Autodesk Fusion 360 part; units mm, degrees
(part 9 of 40)
  line L3796 (254.4894, 100.1276) -> (254.5417, 99.976) construction
  line L3797 (254.5417, 99.976) -> (254.593, 99.8239) construction
  line L3798 (254.593, 99.8239) -> (254.6434, 99.6712) construction
  line L3799 (254.6434, 99.6712) -> (254.6928, 99.518) construction
  line L3800 (254.6928, 99.518) -> (254.7414, 99.3642) construction
  line L3801 (254.7414, 99.3642) -> (254.789, 99.21) construction
  line L3802 (254.789, 99.21) -> (254.8357, 99.0553) construction
  line L3803 (254.8357, 99.0553) -> (254.8815, 98.9001) construction
  line L3804 (254.8815, 98.9001) -> (254.9265, 98.7444) construction
  line L3805 (254.9265, 98.7444) -> (254.9706, 98.5882) construction
  line L3806 (254.9706, 98.5882) -> (255.0138, 98.4316) construction
  line L3807 (255.0138, 98.4316) -> (255.0561, 98.2745) construction
  line L3808 (255.0561, 98.2745) -> (255.0976, 98.117) construction
  line L3809 (255.0976, 98.117) -> (255.1383, 97.9591) construction
  line L3810 (255.1383, 97.9591) -> (255.1781, 97.8007) construction
  line L3811 (255.1781, 97.8007) -> (255.217, 97.6419) construction
  line L3812 (255.217, 97.6419) -> (255.2551, 97.4827) construction
  line L3813 (255.2551, 97.4827) -> (255.2924, 97.3231) construction
  line L3814 (255.2924, 97.3231) -> (255.3289, 97.1631) construction
  line L3815 (255.3289, 97.1631) -> (255.3646, 97.0027) construction
  line L3816 (255.3646, 97.0027) -> (255.3994, 96.8419) construction
  line L3817 (255.3994, 96.8419) -> (255.4335, 96.6807) construction
  line L3818 (255.4335, 96.6807) -> (255.4667, 96.5191) construction
  line L3819 (255.4667, 96.5191) -> (255.4992, 96.3572) construction
  line L3820 (255.4992, 96.3572) -> (255.5308, 96.1949) construction
  line L3821 (255.5308, 96.1949) -> (255.5617, 96.0323) construction
  line L3822 (255.5617, 96.0323) -> (255.5917, 95.8693) construction
  line L3823 (255.5917, 95.8693) -> (255.621, 95.706) construction
  line L3824 (255.621, 95.706) -> (255.6495, 95.5423) construction
  line L3825 (255.6495, 95.5423) -> (255.6773, 95.3783) construction
  line L3826 (255.6773, 95.3783) -> (255.7043, 95.2139) construction
  line L3827 (255.7043, 95.2139) -> (255.7304, 95.0492) construction
  line L3828 (255.7304, 95.0492) -> (255.7559, 94.8842) construction
  line L3829 (255.7559, 94.8842) -> (255.7806, 94.7189) construction
  line L3830 (255.7806, 94.7189) -> (255.8045, 94.5533) construction
  line L3831 (255.8045, 94.5533) -> (255.8276, 94.3874) construction
  line L3832 (255.8276, 94.3874) -> (255.85, 94.2211) construction
  line L3833 (255.85, 94.2211) -> (255.8717, 94.0546) construction
  line L3834 (255.8717, 94.0546) -> (255.8926, 93.8878) construction
  line L3835 (255.8926, 93.8878) -> (255.9087, 93.7541) construction
  line L3836 (255.9087, 93.7541) -> (255.9205, 93.6537) construction
  line L3837 (255.9205, 93.6537) -> (255.9282, 93.5867) construction
  line L3838 (255.9282, 93.5867) -> (255.932, 93.5531) construction
  arc A111 (214.3883, 221.4115) -> (209.8757, 221.4115) centre (212.132, 150) ccw
  arc A112 (262.5041, 122.4018) -> (264.0674, 125.4699) centre (212.132, 150) ccw
  arc A113 (266.6686, 126.4519) -> (264.0674, 125.4699) centre (265.8758, 124.6158) ccw
  arc A114 (266.6686, 126.4519) -> (264.0674, 125.4699) centre (265.8758, 124.6158) ccw
  line L3839 (266.6686, 126.4519) -> (268.1665, 125.8052)
  arc A115 (262.5041, 122.4018) -> (264.0674, 125.4699) centre (212.132, 150) ccw
  line L3840 (266.6686, 126.4519) -> (268.1665, 125.8052)
  arc A116 (262.5041, 122.4018) -> (263.2386, 119.7202) centre (264.2581, 121.4408) ccw
  arc A117 (262.5041, 122.4018) -> (263.2386, 119.7202) centre (264.2581, 121.4408) ccw
  line L3841 (263.2386, 119.7202) -> (264.6423, 118.8885)
  line L3842 (263.2386, 119.7202) -> (264.6423, 118.8885)
  spline S51 degree 5 poles (181.0205, 202.5103) (181.0048, 202.5368) (180.9726, 202.5895) (180.9223, 202.6672) (180.8513, 202.7681) (180.7572, 202.8906) (180.6593, 203.0106) (180.5591, 203.1289) (180.4576, 203.2464) (180.3553, 203.3634) (180.252, 203.4797) (180.1476, 203.5951) (180.0417, 203.7094) (179.9339, 203.8224) (179.8243, 203.934) (179.713, 204.0444) (179.6004, 204.1537) (179.4865, 204.2622) (179.3717, 204.3698) (179.256, 204.4767) (179.1393, 204.5828) (179.0215, 204.6881) (178.9028, 204.7926) (178.7829, 204.8961) (178.662, 204.9988) (178.5401, 205.1007) (178.4172, 205.2017) (178.2934, 205.302) (178.1687, 205.4015) (178.0432, 205.5003) (177.9169, 205.5984) (177.7897, 205.6957) (177.6617, 205.7923) (177.5329, 205.8881) (177.4032, 205.9832) (177.2728, 206.0776) (177.1415, 206.1712) (177.0096, 206.2642) (176.8768, 206.3564) (176.7434, 206.448) (176.6092, 206.5388) (176.4743, 206.629) (176.3387, 206.7185) (176.2025, 206.8073) (176.0655, 206.8955) (175.9278, 206.9829) (175.7895, 207.0697) (175.6505, 207.1558) (175.5109, 207.2413) (175.3706, 207.3261) (175.2297, 207.4102) (175.0882, 207.4937) (174.946, 207.5765) (174.8032, 207.6587) (174.6599, 207.7403) (174.5159, 207.8212) (174.3713, 207.9014) (174.2262, 207.981) (174.0805, 208.06) (173.9342, 208.1383) (173.7873, 208.216) (173.6399, 208.2931) (173.4919, 208.3695) (173.3434, 208.4453) (173.1943, 208.5205) (173.0447, 208.595) (172.8946, 208.669) (172.7439, 208.7423) (172.5927, 208.8149) (172.4411, 208.887) (172.2889, 208.9584) (172.1667, 209.0151) (172.0748, 209.0573) (172.0135, 209.0853) (171.9828, 209.0993) knots 0 0 0 0 0 0 0.01428571 0.02857143 0.04285714 0.05714286 0.07142857 0.08571429 0.1 0.11428571 0.12857143 0.14285714 0.15714286 0.17142857 0.18571429 0.2 0.21428571 0.22857143 0.24285714 0.25714286 0.27142857 0.28571429 0.3 0.31428571 0.32857143 0.34285714 0.35714286 0.37142857 0.38571429 0.4 0.41428571 0.42857143 0.44285714 0.45714286 0.47142857 0.48571429 0.5 0.51428571 0.52857143 0.54285714 0.55714286 0.57142857 0.58571429 0.6 0.61428571 0.62857143 0.64285714 0.65714286 0.67142857 0.68571429 0.7 0.71428571 0.72857143 0.74285714 0.75714286 0.77142857 0.78571429 0.8 0.81428571 0.82857143 0.84285714 0.85714286 0.87142857 0.88571429 0.9 0.91428571 0.92857143 0.94285714 0.95714286 0.97142857 0.98571429 1 1 1 1 1 1
  line L3843 (181.0205, 202.5103) -> (181.0048, 202.5368) construction
  line L3844 (181.0048, 202.5368) -> (180.9726, 202.5895) construction
  line L3845 (180.9726, 202.5895) -> (180.9223, 202.6672) construction
  line L3846 (180.9223, 202.6672) -> (180.8513, 202.7681) construction
  line L3847 (180.8513, 202.7681) -> (180.7572, 202.8906) construction
  line L3848 (180.7572, 202.8906) -> (180.6593, 203.0106) construction
  line L3849 (180.6593, 203.0106) -> (180.5591, 203.1289) construction
  line L3850 (180.5591, 203.1289) -> (180.4576, 203.2464) construction
  line L3851 (180.4576, 203.2464) -> (180.3553, 203.3634) construction
  line L3852 (180.3553, 203.3634) -> (180.252, 203.4797) construction
  line L3853 (180.252, 203.4797) -> (180.1476, 203.5951) construction
  line L3854 (180.1476, 203.5951) -> (180.0417, 203.7094) construction
  line L3855 (180.0417, 203.7094) -> (179.9339, 203.8224) construction
  line L3856 (179.9339, 203.8224) -> (179.8243, 203.934) construction
  line L3857 (179.8243, 203.934) -> (179.713, 204.0444) construction
  line L3858 (179.713, 204.0444) -> (179.6004, 204.1537) construction
  line L3859 (179.6004, 204.1537) -> (179.4865, 204.2622) construction
  line L3860 (179.4865, 204.2622) -> (179.3717, 204.3698) construction
  line L3861 (179.3717, 204.3698) -> (179.256, 204.4767) construction
  line L3862 (179.256, 204.4767) -> (179.1393, 204.5828) construction
  line L3863 (179.1393, 204.5828) -> (179.0215, 204.6881) construction
  line L3864 (179.0215, 204.6881) -> (178.9028, 204.7926) construction
  line L3865 (178.9028, 204.7926) -> (178.7829, 204.8961) construction
  line L3866 (178.7829, 204.8961) -> (178.662, 204.9988) construction
  line L3867 (178.662, 204.9988) -> (178.5401, 205.1007) construction
  line L3868 (178.5401, 205.1007) -> (178.4172, 205.2017) construction
  line L3869 (178.4172, 205.2017) -> (178.2934, 205.302) construction
  line L3870 (178.2934, 205.302) -> (178.1687, 205.4015) construction
  line L3871 (178.1687, 205.4015) -> (178.0432, 205.5003) construction
  line L3872 (178.0432, 205.5003) -> (177.9169, 205.5984) construction
  line L3873 (177.9169, 205.5984) -> (177.7897, 205.6957) construction
  line L3874 (177.7897, 205.6957) -> (177.6617, 205.7923) construction
  line L3875 (177.6617, 205.7923) -> (177.5329, 205.8881) construction
  line L3876 (177.5329, 205.8881) -> (177.4032, 205.9832) construction
  line L3877 (177.4032, 205.9832) -> (177.2728, 206.0776) construction
  line L3878 (177.2728, 206.0776) -> (177.1415, 206.1712) construction
  line L3879 (177.1415, 206.1712) -> (177.0096, 206.2642) construction
  line L3880 (177.0096, 206.2642) -> (176.8768, 206.3564) construction
  line L3881 (176.8768, 206.3564) -> (176.7434, 206.448) construction
  line L3882 (176.7434, 206.448) -> (176.6092, 206.5388) construction
  line L3883 (176.6092, 206.5388) -> (176.4743, 206.629) construction
  line L3884 (176.4743, 206.629) -> (176.3387, 206.7185) construction
  line L3885 (176.3387, 206.7185) -> (176.2025, 206.8073) construction
  line L3886 (176.2025, 206.8073) -> (176.0655, 206.8955) construction
  line L3887 (176.0655, 206.8955) -> (175.9278, 206.9829) construction
  line L3888 (175.9278, 206.9829) -> (175.7895, 207.0697) construction
  line L3889 (175.7895, 207.0697) -> (175.6505, 207.1558) construction
  line L3890 (175.6505, 207.1558) -> (175.5109, 207.2413) construction
  line L3891 (175.5109, 207.2413) -> (175.3706, 207.3261) construction
  line L3892 (175.3706, 207.3261) -> (175.2297, 207.4102) construction
  line L3893 (175.2297, 207.4102) -> (175.0882, 207.4937) construction
  line L3894 (175.0882, 207.4937) -> (174.946, 207.5765) construction
  line L3895 (174.946, 207.5765) -> (174.8032, 207.6587) construction
  line L3896 (174.8032, 207.6587) -> (174.6599, 207.7403) construction
  line L3897 (174.6599, 207.7403) -> (174.5159, 207.8212) construction
  line L3898 (174.5159, 207.8212) -> (174.3713, 207.9014) construction
  line L3899 (174.3713, 207.9014) -> (174.2262, 207.981) construction
  line L3900 (174.2262, 207.981) -> (174.0805, 208.06) construction
  line L3901 (174.0805, 208.06) -> (173.9342, 208.1383) construction
  line L3902 (173.9342, 208.1383) -> (173.7873, 208.216) construction
  line L3903 (173.7873, 208.216) -> (173.6399, 208.2931) construction
  line L3904 (173.6399, 208.2931) -> (173.4919, 208.3695) construction
  line L3905 (173.4919, 208.3695) -> (173.3434, 208.4453) construction
  line L3906 (173.3434, 208.4453) -> (173.1943, 208.5205) construction
  line L3907 (173.1943, 208.5205) -> (173.0447, 208.595) construction
  line L3908 (173.0447, 208.595) -> (172.8946, 208.669) construction
  line L3909 (172.8946, 208.669) -> (172.7439, 208.7423) construction
  line L3910 (172.7439, 208.7423) -> (172.5927, 208.8149) construction
  line L3911 (172.5927, 208.8149) -> (172.4411, 208.887) construction
  line L3912 (172.4411, 208.887) -> (172.2889, 208.9584) construction
  line L3913 (172.2889, 208.9584) -> (172.1667, 209.0151) construction
  line L3914 (172.1667, 209.0151) -> (172.0748, 209.0573) construction
  line L3915 (172.0748, 209.0573) -> (172.0135, 209.0853) construction
  line L3916 (172.0135, 209.0853) -> (171.9828, 209.0993) construction
  spline S52 degree 5 poles (236.3268, 93.9655) (236.3391, 93.9372) (236.3628, 93.8802) (236.396, 93.7938) (236.4359, 93.6771) (236.4798, 93.5289) (236.5193, 93.3792) (236.5561, 93.2286) (236.5915, 93.0774) (236.626, 92.9259) (236.6594, 92.774) (236.6914, 92.6217) (236.7216, 92.4688) (236.7496, 92.3152) (236.7755, 92.1609) (236.7994, 92.006) (236.8217, 91.8506) (236.8425, 91.6948) (236.8621, 91.5386) (236.8805, 91.3821) (236.8978, 91.2253) (236.9138, 91.0682) (236.9285, 90.9107) (236.9418, 90.7529) (236.9538, 90.5947) (236.9645, 90.4362) (236.974, 90.2774) (236.9824, 90.1183) (236.9897, 89.9589) (236.9958, 89.7993) (237.0009, 89.6395) (237.0049, 89.4794) (237.0077, 89.3191) (237.0096, 89.1585) (237.0103, 88.9977) (237.01, 88.8367) (237.0086, 88.6755) (237.0062, 88.5141) (237.0028, 88.3525) (236.9985, 88.1907) (236.9931, 88.0288) (236.9868, 87.8666) (236.9795, 87.7043) (236.9712, 87.5419) (236.962, 87.3793) (236.9519, 87.2165) (236.9408, 87.0536) (236.9287, 86.8905) (236.9158, 86.7273) (236.902, 86.564) (236.8872, 86.4005) (236.8716, 86.2369) (236.855, 86.0732) (236.8376, 85.9094) (236.8193, 85.7455) (236.8001, 85.5815) (236.78, 85.4174) (236.7591, 85.2532) (236.7374, 85.0889) (236.7148, 84.9245) (236.6913, 84.76) (236.667, 84.5954) (236.6418, 84.4308) (236.6159, 84.266) (236.5891, 84.1013) (236.5614, 83.9364) (236.533, 83.7715) (236.5038, 83.6065) (236.4737, 83.4415) (236.4428, 83.2764) (236.4112, 83.1113) (236.3852, 82.9792) (236.3654, 82.8801) (236.352, 82.814) (236.3452, 82.7809) knots 0 0 0 0 0 0 0.01428571 0.02857143 0.04285714 0.05714286 0.07142857 0.08571429 0.1 0.11428571 0.12857143 0.14285714 0.15714286 0.17142857 0.18571429 0.2 0.21428571 0.22857143 0.24285714 0.25714286 0.27142857 0.28571429 0.3 0.31428571 0.32857143 0.34285714 0.35714286 0.37142857 0.38571429 0.4 0.41428571 0.42857143 0.44285714 0.45714286 0.47142857 0.48571429 0.5 0.51428571 0.52857143 0.54285714 0.55714286 0.57142857 0.58571429 0.6 0.61428571 0.62857143 0.64285714 0.65714286 0.67142857 0.68571429 0.7 0.71428571 0.72857143 0.74285714 0.75714286 0.77142857 0.78571429 0.8 0.81428571 0.82857143 0.84285714 0.85714286 0.87142857 0.88571429 0.9 0.91428571 0.92857143 0.94285714 0.95714286 0.97142857 0.98571429 1 1 1 1 1 1
  line L3917 (236.3268, 93.9655) -> (236.3391, 93.9372) construction
  line L3918 (236.3391, 93.9372) -> (236.3628, 93.8802) construction
  line L3919 (236.3628, 93.8802) -> (236.396, 93.7938) construction
  line L3920 (236.396, 93.7938) -> (236.4359, 93.6771) construction
  line L3921 (236.4359, 93.6771) -> (236.4798, 93.5289) construction
  line L3922 (236.4798, 93.5289) -> (236.5193, 93.3792) construction
  line L3923 (236.5193, 93.3792) -> (236.5561, 93.2286) construction
  line L3924 (236.5561, 93.2286) -> (236.5915, 93.0774) construction
  line L3925 (236.5915, 93.0774) -> (236.626, 92.9259) construction
  line L3926 (236.626, 92.9259) -> (236.6594, 92.774) construction
  line L3927 (236.6594, 92.774) -> (236.6914, 92.6217) construction
  line L3928 (236.6914, 92.6217) -> (236.7216, 92.4688) construction
  line L3929 (236.7216, 92.4688) -> (236.7496, 92.3152) construction
  line L3930 (236.7496, 92.3152) -> (236.7755, 92.1609) construction
  line L3931 (236.7755, 92.1609) -> (236.7994, 92.006) construction
  line L3932 (236.7994, 92.006) -> (236.8217, 91.8506) construction
  line L3933 (236.8217, 91.8506) -> (236.8425, 91.6948) construction
  line L3934 (236.8425, 91.6948) -> (236.8621, 91.5386) construction
  line L3935 (236.8621, 91.5386) -> (236.8805, 91.3821) construction
  line L3936 (236.8805, 91.3821) -> (236.8978, 91.2253) construction
  line L3937 (236.8978, 91.2253) -> (236.9138, 91.0682) construction
  line L3938 (236.9138, 91.0682) -> (236.9285, 90.9107) construction
  line L3939 (236.9285, 90.9107) -> (236.9418, 90.7529) construction
  line L3940 (236.9418, 90.7529) -> (236.9538, 90.5947) construction
  line L3941 (236.9538, 90.5947) -> (236.9645, 90.4362) construction
  line L3942 (236.9645, 90.4362) -> (236.974, 90.2774) construction
  line L3943 (236.974, 90.2774) -> (236.9824, 90.1183) construction
  line L3944 (236.9824, 90.1183) -> (236.9897, 89.9589) construction
  line L3945 (236.9897, 89.9589) -> (236.9958, 89.7993) construction
  line L3946 (236.9958, 89.7993) -> (237.0009, 89.6395) construction
  line L3947 (237.0009, 89.6395) -> (237.0049, 89.4794) construction
  line L3948 (237.0049, 89.4794) -> (237.0077, 89.3191) construction
  line L3949 (237.0077, 89.3191) -> (237.0096, 89.1585) construction
  line L3950 (237.0096, 89.1585) -> (237.0103, 88.9977) construction
  line L3951 (237.0103, 88.9977) -> (237.01, 88.8367) construction
  line L3952 (237.01, 88.8367) -> (237.0086, 88.6755) construction
  line L3953 (237.0086, 88.6755) -> (237.0062, 88.5141) construction
  line L3954 (237.0062, 88.5141) -> (237.0028, 88.3525) construction
  line L3955 (237.0028, 88.3525) -> (236.9985, 88.1907) construction
  line L3956 (236.9985, 88.1907) -> (236.9931, 88.0288) construction
  line L3957 (236.9931, 88.0288) -> (236.9868, 87.8666) construction
  line L3958 (236.9868, 87.8666) -> (236.9795, 87.7043) construction
  line L3959 (236.9795, 87.7043) -> (236.9712, 87.5419) construction
  line L3960 (236.9712, 87.5419) -> (236.962, 87.3793) construction
  line L3961 (236.962, 87.3793) -> (236.9519, 87.2165) construction
  line L3962 (236.9519, 87.2165) -> (236.9408, 87.0536) construction
  line L3963 (236.9408, 87.0536) -> (236.9287, 86.8905) construction
  line L3964 (236.9287, 86.8905) -> (236.9158, 86.7273) construction
  line L3965 (236.9158, 86.7273) -> (236.902, 86.564) construction
  line L3966 (236.902, 86.564) -> (236.8872, 86.4005) construction
  line L3967 (236.8872, 86.4005) -> (236.8716, 86.2369) construction
  line L3968 (236.8716, 86.2369) -> (236.855, 86.0732) construction
  line L3969 (236.855, 86.0732) -> (236.8376, 85.9094) construction
  line L3970 (236.8376, 85.9094) -> (236.8193, 85.7455) construction
  line L3971 (236.8193, 85.7455) -> (236.8001, 85.5815) construction
  line L3972 (236.8001, 85.5815) -> (236.78, 85.4174) construction
  line L3973 (236.78, 85.4174) -> (236.7591, 85.2532) construction
  line L3974 (236.7591, 85.2532) -> (236.7374, 85.0889) construction
  line L3975 (236.7374, 85.0889) -> (236.7148, 84.9245) construction
  line L3976 (236.7148, 84.9245) -> (236.6913, 84.76) construction
  line L3977 (236.6913, 84.76) -> (236.667, 84.5954) construction
  line L3978 (236.667, 84.5954) -> (236.6418, 84.4308) construction
  line L3979 (236.6418, 84.4308) -> (236.6159, 84.266) construction
  line L3980 (236.6159, 84.266) -> (236.5891, 84.1013) construction
  line L3981 (236.5891, 84.1013) -> (236.5614, 83.9364) construction
  line L3982 (236.5614, 83.9364) -> (236.533, 83.7715) construction
  line L3983 (236.533, 83.7715) -> (236.5038, 83.6065) construction
  line L3984 (236.5038, 83.6065) -> (236.4737, 83.4415) construction
  line L3985 (236.4737, 83.4415) -> (236.4428, 83.2764) construction
  line L3986 (236.4428, 83.2764) -> (236.4112, 83.1113) construction
  line L3987 (236.4112, 83.1113) -> (236.3852, 82.9792) construction
  line L3988 (236.3852, 82.9792) -> (236.3654, 82.8801) construction
  line L3989 (236.3654, 82.8801) -> (236.352, 82.814) construction
  line L3990 (236.352, 82.814) -> (236.3452, 82.7809) construction
  spline S53 degree 5 poles (272.9005, 155.6951) (272.9313, 155.6979) (272.9929, 155.7029) (273.0853, 155.7078) (273.2086, 155.7097) (273.363, 155.7056) (273.5176, 155.6969) (273.6723, 155.6854) (273.827, 155.6723) (273.9818, 155.6583) (274.1365, 155.6431) (274.2913, 155.6265) (274.446, 155.608) (274.6008, 155.5871) (274.7555, 155.5641) (274.9102, 155.539) (275.0649, 155.5121) (275.2195, 155.4838) (275.3741, 155.4542) (275.5286, 155.4233) (275.6831, 155.3913) (275.8375, 155.3579) (275.9918, 155.3232) (276.146, 155.2871) (276.3002, 155.2497) (276.4542, 155.2109) (276.6082, 155.1709) (276.7621, 155.1297) (276.9159, 155.0873) (277.0696, 155.0439) (277.2232, 154.9993) (277.3767, 154.9536) (277.53, 154.9068) (277.6833, 154.8589) (277.8364, 154.8099) (277.9894, 154.7599) (278.1423, 154.7087) (278.2951, 154.6566) (278.4478, 154.6035) (278.6003, 154.5493) (278.7526, 154.4942) (278.9049, 154.438) (279.057, 154.381) (279.209, 154.3229) (279.3608, 154.2639) (279.5124, 154.2039) (279.664, 154.143) (279.8153, 154.0812) (279.9665, 154.0185) (280.1176, 153.9548) (280.2685, 153.8903) (280.4192, 153.8249) (280.5698, 153.7585) (280.7202, 153.6913) (280.8704, 153.6233) (281.0205, 153.5543) (281.1704, 153.4846) (281.3201, 153.4139) (281.4696, 153.3425) (281.619, 153.2701) (281.7682, 153.197) (281.9172, 153.123) (282.066, 153.0482) (282.2146, 152.9726) (282.3631, 152.8962) (282.5113, 152.819) (282.6594, 152.741) (282.8072, 152.6622) (282.9549, 152.5826) (283.1023, 152.5023) (283.2496, 152.4211) (283.3672, 152.3556) (283.4554, 152.3061) (283.5141, 152.2729) (283.5435, 152.2563) knots 0 0 0 0 0 0 0.01428571 0.02857143 0.04285714 0.05714286 0.07142857 0.08571429 0.1 0.11428571 0.12857143 0.14285714 0.15714286 0.17142857 0.18571429 0.2 0.21428571 0.22857143 0.24285714 0.25714286 0.27142857 0.28571429 0.3 0.31428571 0.32857143 0.34285714 0.35714286 0.37142857 0.38571429 0.4 0.41428571 0.42857143 0.44285714 0.45714286 0.47142857 0.48571429 0.5 0.51428571 0.52857143 0.54285714 0.55714286 0.57142857 0.58571429 0.6 0.61428571 0.62857143 0.64285714 0.65714286 0.67142857 0.68571429 0.7 0.71428571 0.72857143 0.74285714 0.75714286 0.77142857 0.78571429 0.8 0.81428571 0.82857143 0.84285714 0.85714286 0.87142857 0.88571429 0.9 0.91428571 0.92857143 0.94285714 0.95714286 0.97142857 0.98571429 1 1 1 1 1 1
  line L3991 (272.9005, 155.6951) -> (272.9313, 155.6979) construction
  line L3992 (272.9313, 155.6979) -> (272.9929, 155.7029) construction
  line L3993 (272.9929, 155.7029) -> (273.0853, 155.7078) construction
  line L3994 (273.0853, 155.7078) -> (273.2086, 155.7097) construction
  line L3995 (273.2086, 155.7097) -> (273.363, 155.7056) construction
  line L3996 (273.363, 155.7056) -> (273.5176, 155.6969) construction
  line L3997 (273.5176, 155.6969) -> (273.6723, 155.6854) construction
  line L3998 (273.6723, 155.6854) -> (273.827, 155.6723) construction
  line L3999 (273.827, 155.6723) -> (273.9818, 155.6583) construction
  line L4000 (273.9818, 155.6583) -> (274.1365, 155.6431) construction
  line L4001 (274.1365, 155.6431) -> (274.2913, 155.6265) construction
  line L4002 (274.2913, 155.6265) -> (274.446, 155.608) construction
  line L4003 (274.446, 155.608) -> (274.6008, 155.5871) construction
  line L4004 (274.6008, 155.5871) -> (274.7555, 155.5641) construction
  line L4005 (274.7555, 155.5641) -> (274.9102, 155.539) construction
  line L4006 (274.9102, 155.539) -> (275.0649, 155.5121) construction
  line L4007 (275.0649, 155.5121) -> (275.2195, 155.4838) construction
  line L4008 (275.2195, 155.4838) -> (275.3741, 155.4542) construction
  line L4009 (275.3741, 155.4542) -> (275.5286, 155.4233) construction
  line L4010 (275.5286, 155.4233) -> (275.6831, 155.3913) construction
  line L4011 (275.6831, 155.3913) -> (275.8375, 155.3579) construction
  line L4012 (275.8375, 155.3579) -> (275.9918, 155.3232) construction
  line L4013 (275.9918, 155.3232) -> (276.146, 155.2871) construction
  line L4014 (276.146, 155.2871) -> (276.3002, 155.2497) construction
  line L4015 (276.3002, 155.2497) -> (276.4542, 155.2109) construction
  line L4016 (276.4542, 155.2109) -> (276.6082, 155.1709) construction
  line L4017 (276.6082, 155.1709) -> (276.7621, 155.1297) construction
  line L4018 (276.7621, 155.1297) -> (276.9159, 155.0873) construction
  line L4019 (276.9159, 155.0873) -> (277.0696, 155.0439) construction
  line L4020 (277.0696, 155.0439) -> (277.2232, 154.9993) construction
  line L4021 (277.2232, 154.9993) -> (277.3767, 154.9536) construction
  line L4022 (277.3767, 154.9536) -> (277.53, 154.9068) construction
  line L4023 (277.53, 154.9068) -> (277.6833, 154.8589) construction
  line L4024 (277.6833, 154.8589) -> (277.8364, 154.8099) construction
  line L4025 (277.8364, 154.8099) -> (277.9894, 154.7599) construction
  line L4026 (277.9894, 154.7599) -> (278.1423, 154.7087) construction
  line L4027 (278.1423, 154.7087) -> (278.2951, 154.6566) construction
  line L4028 (278.2951, 154.6566) -> (278.4478, 154.6035) construction
  line L4029 (278.4478, 154.6035) -> (278.6003, 154.5493) construction
  line L4030 (278.6003, 154.5493) -> (278.7526, 154.4942) construction
  line L4031 (278.7526, 154.4942) -> (278.9049, 154.438) construction
  line L4032 (278.9049, 154.438) -> (279.057, 154.381) construction
  line L4033 (279.057, 154.381) -> (279.209, 154.3229) construction
  line L4034 (279.209, 154.3229) -> (279.3608, 154.2639) construction
  line L4035 (279.3608, 154.2639) -> (279.5124, 154.2039) construction
  line L4036 (279.5124, 154.2039) -> (279.664, 154.143) construction
  line L4037 (279.664, 154.143) -> (279.8153, 154.0812) construction
  line L4038 (279.8153, 154.0812) -> (279.9665, 154.0185) construction
  line L4039 (279.9665, 154.0185) -> (280.1176, 153.9548) construction
  line L4040 (280.1176, 153.9548) -> (280.2685, 153.8903) construction
  line L4041 (280.2685, 153.8903) -> (280.4192, 153.8249) construction
  line L4042 (280.4192, 153.8249) -> (280.5698, 153.7585) construction
  line L4043 (280.5698, 153.7585) -> (280.7202, 153.6913) construction
  line L4044 (280.7202, 153.6913) -> (280.8704, 153.6233) construction
  line L4045 (280.8704, 153.6233) -> (281.0205, 153.5543) construction
  line L4046 (281.0205, 153.5543) -> (281.1704, 153.4846) construction
  line L4047 (281.1704, 153.4846) -> (281.3201, 153.4139) construction
  line L4048 (281.3201, 153.4139) -> (281.4696, 153.3425) construction
  line L4049 (281.4696, 153.3425) -> (281.619, 153.2701) construction
  line L4050 (281.619, 153.2701) -> (281.7682, 153.197) construction
  line L4051 (281.7682, 153.197) -> (281.9172, 153.123) construction
  line L4052 (281.9172, 153.123) -> (282.066, 153.0482) construction
  line L4053 (282.066, 153.0482) -> (282.2146, 152.9726) construction
  line L4054 (282.2146, 152.9726) -> (282.3631, 152.8962) construction
  line L4055 (282.3631, 152.8962) -> (282.5113, 152.819) construction
  line L4056 (282.5113, 152.819) -> (282.6594, 152.741) construction
  line L4057 (282.6594, 152.741) -> (282.8072, 152.6622) construction
  line L4058 (282.8072, 152.6622) -> (282.9549, 152.5826) construction
  line L4059 (282.9549, 152.5826) -> (283.1023, 152.5023) construction
  line L4060 (283.1023, 152.5023) -> (283.2496, 152.4211) construction
  line L4061 (283.2496, 152.4211) -> (283.3672, 152.3556) construction
  line L4062 (283.3672, 152.3556) -> (283.4554, 152.3061) construction
  line L4063 (283.4554, 152.3061) -> (283.5141, 152.2729) construction
  line L4064 (283.5141, 152.2729) -> (283.5435, 152.2563) construction
  spline S54 degree 5 poles (171.8057, 104.1847) (171.7853, 104.1615) (171.7452, 104.1146) (171.6869, 104.0427) (171.6128, 103.944) (171.5254, 103.8167) (171.4416, 103.6865) (171.36, 103.5546) (171.2796, 103.4218) (171.2, 103.2883) (171.1213, 103.1542) (171.0437, 103.0193) (170.9678, 102.8832) (170.8937, 102.7457) (170.8214, 102.607) (170.7507, 102.4671) (170.6816, 102.3262) (170.6136, 102.1844) (170.5467, 102.0419) (170.4808, 101.8988) (170.416, 101.755) (170.3522, 101.6105) (170.2896, 101.4653) (170.2281, 101.3193) (170.1678, 101.1726) (170.1086, 101.0251) (170.0505, 100.877) (169.9934, 100.7283) (169.9373, 100.579) (169.8821, 100.4291) (169.8279, 100.2786) (169.7746, 100.1276) (169.7223, 99.976) (169.671, 99.8239) (169.6206, 99.6712) (169.5712, 99.518) (169.5226, 99.3642) (169.475, 99.21) (169.4283, 99.0553) (169.3825, 98.9001) (169.3375, 98.7444) (169.2934, 98.5882) (169.2502, 98.4316) (169.2079, 98.2745) (169.1664, 98.117) (169.1257, 97.9591) (169.0859, 97.8007) (169.047, 97.6419) (169.0089, 97.4827) (168.9716, 97.3231) (168.9351, 97.1631) (168.8994, 97.0027) (168.8646, 96.8419) (168.8305, 96.6807) (168.7973, 96.5191) (168.7648, 96.3572) (168.7332, 96.1949) (168.7023, 96.0323) (168.6723, 95.8693) (168.643, 95.706) (168.6145, 95.5423) (168.5867, 95.3783) (168.5597, 95.2139) (168.5336, 95.0492) (168.5081, 94.8842) (168.4834, 94.7189) (168.4595, 94.5533) (168.4364, 94.3874) (168.414, 94.2211) (168.3923, 94.0546) (168.3714, 93.8878) (168.3553, 93.7541) (168.3435, 93.6537) (168.3358, 93.5867) (168.332, 93.5531) knots 0 0 0 0 0 0 0.01428571 0.02857143 0.04285714 0.05714286 0.07142857 0.08571429 0.1 0.11428571 0.12857143 0.14285714 0.15714286 0.17142857 0.18571429 0.2 0.21428571 0.22857143 0.24285714 0.25714286 0.27142857 0.28571429 0.3 0.31428571 0.32857143 0.34285714 0.35714286 0.37142857 0.38571429 0.4 0.41428571 0.42857143 0.44285714 0.45714286 0.47142857 0.48571429 0.5 0.51428571 0.52857143 0.54285714 0.55714286 0.57142857 0.58571429 0.6 0.61428571 0.62857143 0.64285714 0.65714286 0.67142857 0.68571429 0.7 0.71428571 0.72857143 0.74285714 0.75714286 0.77142857 0.78571429 0.8 0.81428571 0.82857143 0.84285714 0.85714286 0.87142857 0.88571429 0.9 0.91428571 0.92857143 0.94285714 0.95714286 0.97142857 0.98571429 1 1 1 1 1 1
  line L4065 (171.8057, 104.1847) -> (171.7853, 104.1615) construction
  line L4066 (171.7853, 104.1615) -> (171.7452, 104.1146) construction
  line L4067 (171.7452, 104.1146) -> (171.6869, 104.0427) construction
  line L4068 (171.6869, 104.0427) -> (171.6128, 103.944) construction
  line L4069 (171.6128, 103.944) -> (171.5254, 103.8167) construction
  line L4070 (171.5254, 103.8167) -> (171.4416, 103.6865) construction
  line L4071 (171.4416, 103.6865) -> (171.36, 103.5546) construction
  line L4072 (171.36, 103.5546) -> (171.2796, 103.4218) construction
  line L4073 (171.2796, 103.4218) -> (171.2, 103.2883) construction
  line L4074 (171.2, 103.2883) -> (171.1213, 103.1542) construction
  line L4075 (171.1213, 103.1542) -> (171.0437, 103.0193) construction
  line L4076 (171.0437, 103.0193) -> (170.9678, 102.8832) construction
  line L4077 (170.9678, 102.8832) -> (170.8937, 102.7457) construction
  line L4078 (170.8937, 102.7457) -> (170.8214, 102.607) construction
  line L4079 (170.8214, 102.607) -> (170.7507, 102.4671) construction
  line L4080 (170.7507, 102.4671) -> (170.6816, 102.3262) construction
  line L4081 (170.6816, 102.3262) -> (170.6136, 102.1844) construction
  line L4082 (170.6136, 102.1844) -> (170.5467, 102.0419) construction
  line L4083 (170.5467, 102.0419) -> (170.4808, 101.8988) construction
  line L4084 (170.4808, 101.8988) -> (170.416, 101.755) construction
  line L4085 (170.416, 101.755) -> (170.3522, 101.6105) construction
  line L4086 (170.3522, 101.6105) -> (170.2896, 101.4653) construction
  line L4087 (170.2896, 101.4653) -> (170.2281, 101.3193) construction
  line L4088 (170.2281, 101.3193) -> (170.1678, 101.1726) construction
  line L4089 (170.1678, 101.1726) -> (170.1086, 101.0251) construction
  line L4090 (170.1086, 101.0251) -> (170.0505, 100.877) construction
  line L4091 (170.0505, 100.877) -> (169.9934, 100.7283) construction
  line L4092 (169.9934, 100.7283) -> (169.9373, 100.579) construction
  line L4093 (169.9373, 100.579) -> (169.8821, 100.4291) construction
  line L4094 (169.8821, 100.4291) -> (169.8279, 100.2786) construction
  line L4095 (169.8279, 100.2786) -> (169.7746, 100.1276) construction
  line L4096 (169.7746, 100.1276) -> (169.7223, 99.976) construction
  line L4097 (169.7223, 99.976) -> (169.671, 99.8239) construction
  line L4098 (169.671, 99.8239) -> (169.6206, 99.6712) construction
  line L4099 (169.6206, 99.6712) -> (169.5712, 99.518) construction
  line L4100 (169.5712, 99.518) -> (169.5226, 99.3642) construction
  line L4101 (169.5226, 99.3642) -> (169.475, 99.21) construction
  line L4102 (169.475, 99.21) -> (169.4283, 99.0553) construction
  line L4103 (169.4283, 99.0553) -> (169.3825, 98.9001) construction
  line L4104 (169.3825, 98.9001) -> (169.3375, 98.7444) construction
  line L4105 (169.3375, 98.7444) -> (169.2934, 98.5882) construction
  line L4106 (169.2934, 98.5882) -> (169.2502, 98.4316) construction
  line L4107 (169.2502, 98.4316) -> (169.2079, 98.2745) construction
  line L4108 (169.2079, 98.2745) -> (169.1664, 98.117) construction
  line L4109 (169.1664, 98.117) -> (169.1257, 97.9591) construction
  line L4110 (169.1257, 97.9591) -> (169.0859, 97.8007) construction
  line L4111 (169.0859, 97.8007) -> (169.047, 97.6419) construction
  line L4112 (169.047, 97.6419) -> (169.0089, 97.4827) construction
  line L4113 (169.0089, 97.4827) -> (168.9716, 97.3231) construction
  line L4114 (168.9716, 97.3231) -> (168.9351, 97.1631) construction
  line L4115 (168.9351, 97.1631) -> (168.8994, 97.0027) construction
  line L4116 (168.8994, 97.0027) -> (168.8646, 96.8419) construction
  line L4117 (168.8646, 96.8419) -> (168.8305, 96.6807) construction
  line L4118 (168.8305, 96.6807) -> (168.7973, 96.5191) construction
  line L4119 (168.7973, 96.5191) -> (168.7648, 96.3572) construction
  line L4120 (168.7648, 96.3572) -> (168.7332, 96.1949) construction
  line L4121 (168.7332, 96.1949) -> (168.7023, 96.0323) construction
  line L4122 (168.7023, 96.0323) -> (168.6723, 95.8693) construction
  line L4123 (168.6723, 95.8693) -> (168.643, 95.706) construction
  line L4124 (168.643, 95.706) -> (168.6145, 95.5423) construction
  line L4125 (168.6145, 95.5423) -> (168.5867, 95.3783) construction
  line L4126 (168.5867, 95.3783) -> (168.5597, 95.2139) construction
  line L4127 (168.5597, 95.2139) -> (168.5336, 95.0492) construction
  line L4128 (168.5336, 95.0492) -> (168.5081, 94.8842) construction
  line L4129 (168.5081, 94.8842) -> (168.4834, 94.7189) construction
  line L4130 (168.4834, 94.7189) -> (168.4595, 94.5533) construction
  line L4131 (168.4595, 94.5533) -> (168.4364, 94.3874) construction
  line L4132 (168.4364, 94.3874) -> (168.414, 94.2211) construction
  line L4133 (168.414, 94.2211) -> (168.3923, 94.0546) construction
  line L4134 (168.3923, 94.0546) -> (168.3714, 93.8878) construction
  line L4135 (168.3714, 93.8878) -> (168.3553, 93.7541) construction
  line L4136 (168.3553, 93.7541) -> (168.3435, 93.6537) construction
  line L4137 (168.3435, 93.6537) -> (168.3358, 93.5867) construction
  line L4138 (168.3358, 93.5867) -> (168.332, 93.5531) construction
  arc A118 (283.5435, 147.7437) -> (283.5435, 152.2563) centre (212.132, 150) ccw
  arc A119 (252.2812, 90.9007) -> (255.932, 93.5531) centre (212.132, 150) ccw
  arc A120 (232.0535, 81.3864) -> (236.3452, 82.7809) centre (212.132, 150) ccw
  arc A121 (232.0535, 81.3864) -> (236.3452, 82.7809) centre (212.132, 150) ccw
  spline S55 degree 5 poles (236.3268, 93.9655) (236.3391, 93.9372) (236.3628, 93.8802) (236.396, 93.7938) (236.4359, 93.6771) (236.4798, 93.5289) (236.5193, 93.3792) (236.5561, 93.2286) (236.5915, 93.0774) (236.626, 92.9259) (236.6594, 92.774) (236.6914, 92.6217) (236.7216, 92.4688) (236.7496, 92.3152) (236.7755, 92.1609) (236.7994, 92.006) (236.8217, 91.8506) (236.8425, 91.6948) (236.8621, 91.5386) (236.8805, 91.3821) (236.8978, 91.2253) (236.9138, 91.0682) (236.9285, 90.9107) (236.9418, 90.7529) (236.9538, 90.5947) (236.9645, 90.4362) (236.974, 90.2774) (236.9824, 90.1183) (236.9897, 89.9589) (236.9958, 89.7993) (237.0009, 89.6395) (237.0049, 89.4794) (237.0077, 89.3191) (237.0096, 89.1585) (237.0103, 88.9977) (237.01, 88.8367) (237.0086, 88.6755) (237.0062, 88.5141) (237.0028, 88.3525) (236.9985, 88.1907) (236.9931, 88.0288) (236.9868, 87.8666) (236.9795, 87.7043) (236.9712, 87.5419) (236.962, 87.3793) (236.9519, 87.2165) (236.9408, 87.0536) (236.9287, 86.8905) (236.9158, 86.7273) (236.902, 86.564) (236.8872, 86.4005) (236.8716, 86.2369) (236.855, 86.0732) (236.8376, 85.9094) (236.8193, 85.7455) (236.8001, 85.5815) (236.78, 85.4174) (236.7591, 85.2532) (236.7374, 85.0889) (236.7148, 84.9245) (236.6913, 84.76) (236.667, 84.5954) (236.6418, 84.4308) (236.6159, 84.266) (236.5891, 84.1013) (236.5614, 83.9364) (236.533, 83.7715) (236.5038, 83.6065) (236.4737, 83.4415) (236.4428, 83.2764) (236.4112, 83.1113) (236.3852, 82.9792) (236.3654, 82.8801) (236.352, 82.814) (236.3452, 82.7809) knots 0 0 0 0 0 0 0.01428571 0.02857143 0.04285714 0.05714286 0.07142857 0.08571429 0.1 0.11428571 0.12857143 0.14285714 0.15714286 0.17142857 0.18571429 0.2 0.21428571 0.22857143 0.24285714 0.25714286 0.27142857 0.28571429 0.3 0.31428571 0.32857143 0.34285714 0.35714286 0.37142857 0.38571429 0.4 0.41428571 0.42857143 0.44285714 0.45714286 0.47142857 0.48571429 0.5 0.51428571 0.52857143 0.54285714 0.55714286 0.57142857 0.58571429 0.6 0.61428571 0.62857143 0.64285714 0.65714286 0.67142857 0.68571429 0.7 0.71428571 0.72857143 0.74285714 0.75714286 0.77142857 0.78571429 0.8 0.81428571 0.82857143 0.84285714 0.85714286 0.87142857 0.88571429 0.9 0.91428571 0.92857143 0.94285714 0.95714286 0.97142857 0.98571429 1 1 1 1 1 1
  line L4139 (236.3268, 93.9655) -> (236.3391, 93.9372) construction
  line L4140 (236.3391, 93.9372) -> (236.3628, 93.8802) construction
  line L4141 (236.3628, 93.8802) -> (236.396, 93.7938) construction
  line L4142 (236.396, 93.7938) -> (236.4359, 93.6771) construction
  line L4143 (236.4359, 93.6771) -> (236.4798, 93.5289) construction
  line L4144 (236.4798, 93.5289) -> (236.5193, 93.3792) construction
  line L4145 (236.5193, 93.3792) -> (236.5561, 93.2286) construction
  line L4146 (236.5561, 93.2286) -> (236.5915, 93.0774) construction
  line L4147 (236.5915, 93.0774) -> (236.626, 92.9259) construction
  line L4148 (236.626, 92.9259) -> (236.6594, 92.774) construction
  line L4149 (236.6594, 92.774) -> (236.6914, 92.6217) construction
  line L4150 (236.6914, 92.6217) -> (236.7216, 92.4688) construction
  line L4151 (236.7216, 92.4688) -> (236.7496, 92.3152) construction
  line L4152 (236.7496, 92.3152) -> (236.7755, 92.1609) construction
  line L4153 (236.7755, 92.1609) -> (236.7994, 92.006) construction
  line L4154 (236.7994, 92.006) -> (236.8217, 91.8506) construction
  line L4155 (236.8217, 91.8506) -> (236.8425, 91.6948) construction
  line L4156 (236.8425, 91.6948) -> (236.8621, 91.5386) construction
  line L4157 (236.8621, 91.5386) -> (236.8805, 91.3821) construction
  line L4158 (236.8805, 91.3821) -> (236.8978, 91.2253) construction
  line L4159 (236.8978, 91.2253) -> (236.9138, 91.0682) construction
  line L4160 (236.9138, 91.0682) -> (236.9285, 90.9107) construction
  line L4161 (236.9285, 90.9107) -> (236.9418, 90.7529) construction
  line L4162 (236.9418, 90.7529) -> (236.9538, 90.5947) construction
  line L4163 (236.9538, 90.5947) -> (236.9645, 90.4362) construction
  line L4164 (236.9645, 90.4362) -> (236.974, 90.2774) construction
  line L4165 (236.974, 90.2774) -> (236.9824, 90.1183) construction
  line L4166 (236.9824, 90.1183) -> (236.9897, 89.9589) construction
  line L4167 (236.9897, 89.9589) -> (236.9958, 89.7993) construction
  line L4168 (236.9958, 89.7993) -> (237.0009, 89.6395) construction
  line L4169 (237.0009, 89.6395) -> (237.0049, 89.4794) construction
  line L4170 (237.0049, 89.4794) -> (237.0077, 89.3191) construction
  line L4171 (237.0077, 89.3191) -> (237.0096, 89.1585) construction
  line L4172 (237.0096, 89.1585) -> (237.0103, 88.9977) construction
  line L4173 (237.0103, 88.9977) -> (237.01, 88.8367) construction
  line L4174 (237.01, 88.8367) -> (237.0086, 88.6755) construction
  line L4175 (237.0086, 88.6755) -> (237.0062, 88.5141) construction
  line L4176 (237.0062, 88.5141) -> (237.0028, 88.3525) construction
  line L4177 (237.0028, 88.3525) -> (236.9985, 88.1907) construction
  line L4178 (236.9985, 88.1907) -> (236.9931, 88.0288) construction
  line L4179 (236.9931, 88.0288) -> (236.9868, 87.8666) construction
  line L4180 (236.9868, 87.8666) -> (236.9795, 87.7043) construction
  line L4181 (236.9795, 87.7043) -> (236.9712, 87.5419) construction
  line L4182 (236.9712, 87.5419) -> (236.962, 87.3793) construction
  line L4183 (236.962, 87.3793) -> (236.9519, 87.2165) construction
  line L4184 (236.9519, 87.2165) -> (236.9408, 87.0536) construction
  line L4185 (236.9408, 87.0536) -> (236.9287, 86.8905) construction
  line L4186 (236.9287, 86.8905) -> (236.9158, 86.7273) construction
  line L4187 (236.9158, 86.7273) -> (236.902, 86.564) construction
  line L4188 (236.902, 86.564) -> (236.8872, 86.4005) construction
  line L4189 (236.8872, 86.4005) -> (236.8716, 86.2369) construction
  line L4190 (236.8716, 86.2369) -> (236.855, 86.0732) construction
  line L4191 (236.855, 86.0732) -> (236.8376, 85.9094) construction
  line L4192 (236.8376, 85.9094) -> (236.8193, 85.7455) construction
  line L4193 (236.8193, 85.7455) -> (236.8001, 85.5815) construction
  line L4194 (236.8001, 85.5815) -> (236.78, 85.4174) construction
  line L4195 (236.78, 85.4174) -> (236.7591, 85.2532) construction
  line L4196 (236.7591, 85.2532) -> (236.7374, 85.0889) construction
  line L4197 (236.7374, 85.0889) -> (236.7148, 84.9245) construction
  line L4198 (236.7148, 84.9245) -> (236.6913, 84.76) construction
  line L4199 (236.6913, 84.76) -> (236.667, 84.5954) construction
  line L4200 (236.667, 84.5954) -> (236.6418, 84.4308) construction
  line L4201 (236.6418, 84.4308) -> (236.6159, 84.266) construction
  line L4202 (236.6159, 84.266) -> (236.5891, 84.1013) construction
  line L4203 (236.5891, 84.1013) -> (236.5614, 83.9364) construction
  line L4204 (236.5614, 83.9364) -> (236.533, 83.7715) construction
  line L4205 (236.533, 83.7715) -> (236.5038, 83.6065) construction
  line L4206 (236.5038, 83.6065) -> (236.4737, 83.4415) construction
  line L4207 (236.4737, 83.4415) -> (236.4428, 83.2764) construction
  line L4208 (236.4428, 83.2764) -> (236.4112, 83.1113) construction
  line L4209 (236.4112, 83.1113) -> (236.3852, 82.9792) construction
  line L4210 (236.3852, 82.9792) -> (236.3654, 82.8801) construction
  line L4211 (236.3654, 82.8801) -> (236.352, 82.814) construction
  line L4212 (236.352, 82.814) -> (236.3452, 82.7809) construction
  arc A122 (168.332, 93.5531) -> (171.9828, 90.9007) centre (212.132, 150) ccw
  arc A123 (252.2812, 90.9007) -> (255.932, 93.5531) centre (212.132, 150) ccw
  arc A124 (168.332, 93.5531) -> (171.9828, 90.9007) centre (212.132, 150) ccw
  spline S56 degree 5 poles (181.0205, 97.4897) (181.0048, 97.4632) (180.9726, 97.4105) (180.9223, 97.3328) (180.8513, 97.2319) (180.7572, 97.1094) (180.6593, 96.9894) (180.5591, 96.8711) (180.4576, 96.7536) (180.3553, 96.6366) (180.252, 96.5203) (180.1476, 96.4049) (180.0417, 96.2906) (179.9339, 96.1776) (179.8243, 96.066) (179.713, 95.9556) (179.6004, 95.8463) (179.4865, 95.7378) (179.3717, 95.6302) (179.256, 95.5233) (179.1393, 95.4172) (179.0215, 95.3119) (178.9028, 95.2074) (178.7829, 95.1039) (178.662, 95.0012) (178.5401, 94.8993) (178.4172, 94.7983) (178.2934, 94.698) (178.1687, 94.5985) (178.0432, 94.4997) (177.9169, 94.4016) (177.7897, 94.3043) (177.6617, 94.2077) (177.5329, 94.1119) (177.4032, 94.0168) (177.2728, 93.9224) (177.1415, 93.8288) (177.0096, 93.7358) (176.8768, 93.6436) (176.7434, 93.552) (176.6092, 93.4612) (176.4743, 93.371) (176.3387, 93.2815) (176.2025, 93.1927) (176.0655, 93.1045) (175.9278, 93.0171) (175.7895, 92.9303) (175.6505, 92.8442) (175.5109, 92.7587) (175.3706, 92.6739) (175.2297, 92.5898) (175.0882, 92.5063) (174.946, 92.4235) (174.8032, 92.3413) (174.6599, 92.2597) (174.5159, 92.1788) (174.3713, 92.0986) (174.2262, 92.019) (174.0805, 91.94) (173.9342, 91.8617) (173.7873, 91.784) (173.6399, 91.7069) (173.4919, 91.6305) (173.3434, 91.5547) (173.1943, 91.4795) (173.0447, 91.405) (172.8946, 91.331) (172.7439, 91.2577) (172.5927, 91.1851) (172.4411, 91.113) (172.2889, 91.0416) (172.1667, 90.9849) (172.0748, 90.9427) (172.0135, 90.9147) (171.9828, 90.9007) knots 0 0 0 0 0 0 0.01428571 0.02857143 0.04285714 0.05714286 0.07142857 0.08571429 0.1 0.11428571 0.12857143 0.14285714 0.15714286 0.17142857 0.18571429 0.2 0.21428571 0.22857143 0.24285714 0.25714286 0.27142857 0.28571429 0.3 0.31428571 0.32857143 0.34285714 0.35714286 0.37142857 0.38571429 0.4 0.41428571 0.42857143 0.44285714 0.45714286 0.47142857 0.48571429 0.5 0.51428571 0.52857143 0.54285714 0.55714286 0.57142857 0.58571429 0.6 0.61428571 0.62857143 0.64285714 0.65714286 0.67142857 0.68571429 0.7 0.71428571 0.72857143 0.74285714 0.75714286 0.77142857 0.78571429 0.8 0.81428571 0.82857143 0.84285714 0.85714286 0.87142857 0.88571429 0.9 0.91428571 0.92857143 0.94285714 0.95714286 0.97142857 0.98571429 1 1 1 1 1 1
  line L4213 (181.0205, 97.4897) -> (181.0048, 97.4632) construction
  line L4214 (181.0048, 97.4632) -> (180.9726, 97.4105) construction
  line L4215 (180.9726, 97.4105) -> (180.9223, 97.3328) construction
  line L4216 (180.9223, 97.3328) -> (180.8513, 97.2319) construction
  line L4217 (180.8513, 97.2319) -> (180.7572, 97.1094) construction
  line L4218 (180.7572, 97.1094) -> (180.6593, 96.9894) construction
  line L4219 (180.6593, 96.9894) -> (180.5591, 96.8711) construction
  line L4220 (180.5591, 96.8711) -> (180.4576, 96.7536) construction
  line L4221 (180.4576, 96.7536) -> (180.3553, 96.6366) construction
  line L4222 (180.3553, 96.6366) -> (180.252, 96.5203) construction
  line L4223 (180.252, 96.5203) -> (180.1476, 96.4049) construction
  line L4224 (180.1476, 96.4049) -> (180.0417, 96.2906) construction
  line L4225 (180.0417, 96.2906) -> (179.9339, 96.1776) construction
  line L4226 (179.9339, 96.1776) -> (179.8243, 96.066) construction
  line L4227 (179.8243, 96.066) -> (179.713, 95.9556) construction
  line L4228 (179.713, 95.9556) -> (179.6004, 95.8463) construction
  line L4229 (179.6004, 95.8463) -> (179.4865, 95.7378) construction
  line L4230 (179.4865, 95.7378) -> (179.3717, 95.6302) construction
  line L4231 (179.3717, 95.6302) -> (179.256, 95.5233) construction
  line L4232 (179.256, 95.5233) -> (179.1393, 95.4172) construction
  line L4233 (179.1393, 95.4172) -> (179.0215, 95.3119) construction
  line L4234 (179.0215, 95.3119) -> (178.9028, 95.2074) construction
  line L4235 (178.9028, 95.2074) -> (178.7829, 95.1039) construction
  line L4236 (178.7829, 95.1039) -> (178.662, 95.0012) construction
  line L4237 (178.662, 95.0012) -> (178.5401, 94.8993) construction
  line L4238 (178.5401, 94.8993) -> (178.4172, 94.7983) construction
  line L4239 (178.4172, 94.7983) -> (178.2934, 94.698) construction
  line L4240 (178.2934, 94.698) -> (178.1687, 94.5985) construction
  line L4241 (178.1687, 94.5985) -> (178.0432, 94.4997) construction
  line L4242 (178.0432, 94.4997) -> (177.9169, 94.4016) construction
  line L4243 (177.9169, 94.4016) -> (177.7897, 94.3043) construction
  line L4244 (177.7897, 94.3043) -> (177.6617, 94.2077) construction
  line L4245 (177.6617, 94.2077) -> (177.5329, 94.1119) construction
  line L4246 (177.5329, 94.1119) -> (177.4032, 94.0168) construction
  line L4247 (177.4032, 94.0168) -> (177.2728, 93.9224) construction
  line L4248 (177.2728, 93.9224) -> (177.1415, 93.8288) construction
  line L4249 (177.1415, 93.8288) -> (177.0096, 93.7358) construction
  line L4250 (177.0096, 93.7358) -> (176.8768, 93.6436) construction
  line L4251 (176.8768, 93.6436) -> (176.7434, 93.552) construction
  line L4252 (176.7434, 93.552) -> (176.6092, 93.4612) construction
  line L4253 (176.6092, 93.4612) -> (176.4743, 93.371) construction
  line L4254 (176.4743, 93.371) -> (176.3387, 93.2815) construction
  line L4255 (176.3387, 93.2815) -> (176.2025, 93.1927) construction
  line L4256 (176.2025, 93.1927) -> (176.0655, 93.1045) construction
  line L4257 (176.0655, 93.1045) -> (175.9278, 93.0171) construction
  line L4258 (175.9278, 93.0171) -> (175.7895, 92.9303) construction
  line L4259 (175.7895, 92.9303) -> (175.6505, 92.8442) construction
  line L4260 (175.6505, 92.8442) -> (175.5109, 92.7587) construction
  line L4261 (175.5109, 92.7587) -> (175.3706, 92.6739) construction
  line L4262 (175.3706, 92.6739) -> (175.2297, 92.5898) construction
  line L4263 (175.2297, 92.5898) -> (175.0882, 92.5063) construction
  line L4264 (175.0882, 92.5063) -> (174.946, 92.4235) construction
  line L4265 (174.946, 92.4235) -> (174.8032, 92.3413) construction
  line L4266 (174.8032, 92.3413) -> (174.6599, 92.2597) construction
  line L4267 (174.6599, 92.2597) -> (174.5159, 92.1788) construction
  line L4268 (174.5159, 92.1788) -> (174.3713, 92.0986) construction
  line L4269 (174.3713, 92.0986) -> (174.2262, 92.019) construction
  line L4270 (174.2262, 92.019) -> (174.0805, 91.94) construction
  line L4271 (174.0805, 91.94) -> (173.9342, 91.8617) construction
  line L4272 (173.9342, 91.8617) -> (173.7873, 91.784) construction
  line L4273 (173.7873, 91.784) -> (173.6399, 91.7069) construction
  line L4274 (173.6399, 91.7069) -> (173.4919, 91.6305) construction
  line L4275 (173.4919, 91.6305) -> (173.3434, 91.5547) construction
  line L4276 (173.3434, 91.5547) -> (173.1943, 91.4795) construction
  line L4277 (173.1943, 91.4795) -> (173.0447, 91.405) construction
  line L4278 (173.0447, 91.405) -> (172.8946, 91.331) construction
  line L4279 (172.8946, 91.331) -> (172.7439, 91.2577) construction
  line L4280 (172.7439, 91.2577) -> (172.5927, 91.1851) construction
  line L4281 (172.5927, 91.1851) -> (172.4411, 91.113) construction
  line L4282 (172.4411, 91.113) -> (172.2889, 91.0416) construction
  line L4283 (172.2889, 91.0416) -> (172.1667, 90.9849) construction
  line L4284 (172.1667, 90.9849) -> (172.0748, 90.9427) construction
  line L4285 (172.0748, 90.9427) -> (172.0135, 90.9147) construction
  line L4286 (172.0135, 90.9147) -> (171.9828, 90.9007) construction